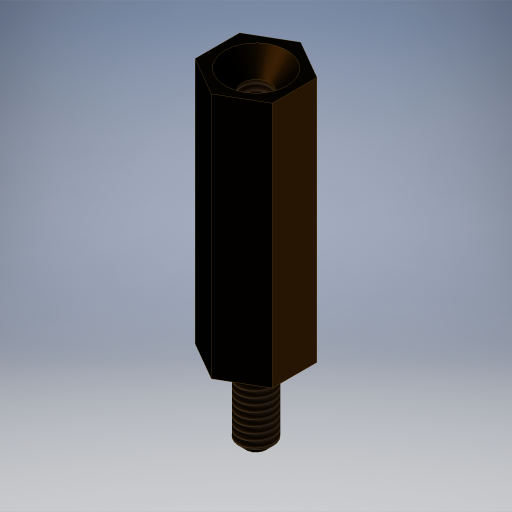
# Autodesk Inventor part: 2.5x18mm Standoff
Saved by Autodesk Inventor 2024 (Build 280153000, 153)
## iProperties
Created: 2024-11-19
Part Number: 2.5x18mm Standoff
Material: Bronze, Soft Tin
Document SubType Name: Modeling
Designer: Stefano
Density: 8.874 g/cm^3
Appearance: Brass - Satin
Author: Stefano
Autodesk Inventor part; units mm, degrees
ref_plane "YZ Plane" through (0, 0, 0) normal (1, 0, 0) x (0, 1, 0)
ref_plane "XZ Plane" through (0, 0, 0) normal (0, 1, 0) x (-1, 0, 0)
ref_plane "XY Plane" through (0, 0, 0) normal (0, 0, 1) x (1, 0, 0)
sketch "Sketch1" plane through (0, 0, 0) normal (0, 1, 0) x (-1, 0, 0)
  line L0 (0, 3.2563) -> (2.82, 1.6281)
  line L1 (2.82, 1.6281) -> (2.82, -1.6281)
  line L2 (2.82, -1.6281) -> (0, -3.2563)
  line L3 (0, -3.2563) -> (-2.82, -1.6281)
  line L4 (-2.82, -1.6281) -> (-2.82, 1.6281)
  line L5 (-2.82, 1.6281) -> (0, 3.2563)
  point P0 (0, 0)
  point P1 (0, 0)
  dimension "d0" = 5.64
  constraints: 12 end point, 1 coincident, 13 other
  measures "d0" distance between parallel lines of L4 L1
extrude "Extrusion1" add sketch "Sketch1" along normal blind 18
sketch "Sketch2" plane through (0, 18, 0) normal (0, 1, 0) x (1, 0, 0)
  point P0 (0, 0)
  point P1 (0, 0)
  constraints: 1 coincident
hole "Hole1" at (0, 18, 0) direction (0, -1, 0) diameter 2.013 depth 7.6 tip angle 118 countersink diameter 4.5 countersink angle 82 thread size "M2.5x0.45" class "6H" standard "ANSI Metric M Profile"
sketch "Sketch3" plane through (0, 0, 0) normal (0, -1, 0) x (1, 0, 0)
  circle A0 centre (0, 0) radius 1.25
  dimension "d10" = 2.5
  constraints: 1 centre point, 1 coincident
  measures "d10" diameter of A0
extrude "Extrusion2" add sketch "Sketch3" along normal blind 5.75
thread "Thread1" size "M2.5x0.45" class "6g" standard "ANSI Metric M Profile" full length
chamfer "Chamfer1" distance 0.5 angle 45 1 edges at (-1.25, -5.75, 0)
body "Solid1"
